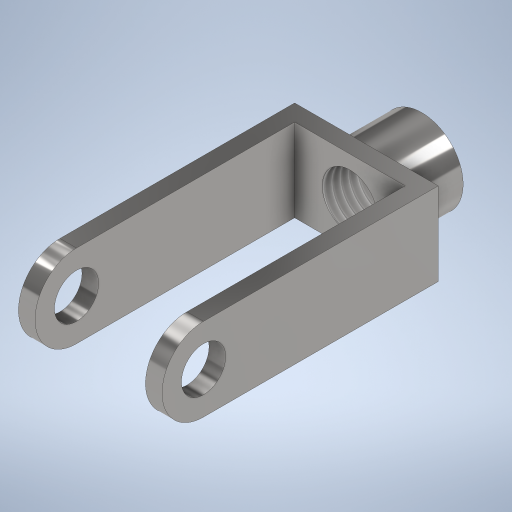
# Autodesk Inventor part: ustück
Saved by Autodesk Inventor 2024.4 (Build 284460000, 460)
## iProperties
Created: 2026-01-12
Part Number: ustück
Material: Stahl
Document SubType Name: Modeling
Designer: PC
Density: 7.85 g/cm^3
Appearance: Stahl - poliert
Description: UStück
Mass: 46.9601 g
Surface Area: 51.3116 cm^2
Volume: 5.98217 cm^3
Masse[kg]: 0,047 kg
Autodesk Inventor part; units mm, degrees
ref_plane "YZ Plane" through (0, 0, 0) normal (1, 0, 0) x (0, 1, 0)
ref_plane "XZ Plane" through (0, 0, 0) normal (0, 1, 0) x (-1, 0, 0)
ref_plane "XY Plane" through (0, 0, 0) normal (0, 0, 1) x (1, 0, 0)
sketch "Skizze1" plane through (0, 0, 0) normal (0, 0, 1) x (1, 0, 0)
  line L0 (0, 0) -> (-13, 0)
  line L1 (-13, 0) -> (-13, -50)
  line L2 (-13, -50) -> (-10, -50)
  line L3 (-10, -50) -> (-10, -3)
  line L4 (-10, -3) -> (0, -3)
  line L5 (0, -3) -> (0, 0)
  line L6 (-13, 0) -> (0, 0)
  line L7 (0, 10) -> (0, -60) projected
  line L8 (0, 0) -> (13, 0)
  line L9 (13, 0) -> (13, -50)
  line L10 (13, -50) -> (10, -50)
  line L11 (10, -50) -> (10, -3)
  line L12 (10, -3) -> (0, -3)
  line L13 (13, 0) -> (0, 0)
  dimension "d0" = 13
  dimension "d1" = 50
  dimension "d2" = 3
  dimension "d3" = 47
  constraints: 26 end point, 4 symmetric about line, 3 perpendicular, 1 collinear, 1 horizontal, 1 parallel, 1 vertical
  measures "d0" distance of L0.start L0.end
  measures "d1" distance of L0.end L1.end
  measures "d2" distance of L1.end L2.end
  measures "d3" distance of L2.end L3.end
extrude "Extrusion1" add sketch "Skizze1" along normal mid plane 15
sketch "Skizze2" plane through (-13, -50, 7.5) normal (-1, 0, 0) x (0, 0, 1)
  line L0 (-15, 0) -> (-15, 50) projected
  line L1 (-15, 0) -> (0, 0) projected
  line L2 (-15, 50) -> (0, 50)
  line L3 (0, 50) -> (0, 7.5)
  line L4 (-7.5, 0) -> (-7.5, 0)
  line L5 (-15, 7.5) -> (-15, 50)
  arc A0 (-15, 7.5) -> (-7.5, 0) centre (-7.5, 7.5) ccw
  arc A1 (-7.5, 0) -> (0, 7.5) centre (-7.5, 7.5) ccw
  circle A2 centre (-7.5, 7.5) radius 4
  line L6 (-15, 50) -> (0, 50)
  line L7 (0, 50) -> (0, 0)
  line L8 (0, 0) -> (-15, 0)
  line L9 (-15, 0) -> (-15, 50)
  point P0 (-7.5, 50)
  point P1 (0, 7.5)
  point P2 (-7.5, 0)
  point P3 (-7.5, 0)
  point P4 (-7.5, 0)
  point P5 (-15, 7.5)
  dimension "d6" = 7.5
  dimension "d7" = 8
  constraints: 16 end point, 4 parallel, 4 point on circle, 4 tangent, 3 centre point, 2 horizontal, 2 perpendicular, 2 point on line, 1 coincident, 1 concentric
  measures "d6" radius of A0
  measures "d7" diameter of A2
extrude "Extrusion2" cut sketch "Skizze2" against normal through all contours L0 A0 L1 | A1 L7 L1 | A2
sketch "Skizze3" plane through (-13, 0, 7.5) normal (0, 1, 0) x (1, 0, 0)
  circle A0 centre (13, 7.5) radius 5
  dimension "d10" = 10
  constraints: 1 centre point, 1 coincident
  measures "d10" diameter of A0
extrude "Extrusion3" cut sketch "Skizze3" against normal through all
sketch "Skizze4" plane through (-13, 0, 7.5) normal (0, 1, 0) x (1, 0, 0)
  circle A0 centre (13, 7.5) radius 5 projected
  circle A1 centre (13, 7.5) radius 5
  circle A2 centre (13, 7.5) radius 7.5
  dimension "d13" = 2.5
  constraints: 2 centre point, 1 coincident
  measures "d13" radial gap between concentric circles of A0 A2
extrude "Extrusion4" add sketch "Skizze4" along normal blind 10
thread "Gewinde1" size "M10x1.5" class "6H" standard "ANSI Metric M Profile" full length
